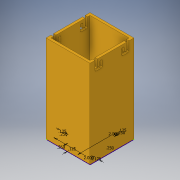
# Autodesk Inventor part: bateryHolder2.0
Saved by Autodesk Inventor 2017 (Build 210142000, 142)
## iProperties
Created: 2018-01-06
Part Number: bateryHolder2.0
Material: Generic
Document SubType Name: Modeling
Designer: User
Density: 1 g/cm^3
Appearance: Default(1)
Author: User
Autodesk Inventor part; units mm, degrees
ref_plane "YZ Plane" through (0, 0, 0) normal (1, 0, 0) x (0, 1, 0)
ref_plane "XZ Plane" through (0, 0, 0) normal (0, 1, 0) x (-1, 0, 0)
ref_plane "XY Plane" through (0, 0, 0) normal (0, 0, 1) x (1, 0, 0)
sketch "Sketch1" plane through (0, 0, 0) normal (0, 1, 0) x (-1, 0, 0)
  line L0 (0, 0) -> (50.8, 0)
  line L1 (50.8, 0) -> (50.8, -50.8)
  line L2 (50.8, -50.8) -> (0, -50.8)
  line L3 (0, -50.8) -> (0, 0)
  line L4 (53.975, 0) -> (53.975, 3.175)
  line L5 (53.975, 3.175) -> (50.8, 3.175)
  line L6 (-3.175, -50.8) -> (-3.175, -53.975)
  line L7 (-3.175, -53.975) -> (0, -53.975)
  line L8 (-3.175, -53.975) -> (53.975, -53.975)
  line L9 (53.975, -53.975) -> (53.975, 3.175)
  line L10 (53.975, 3.175) -> (-3.175, 3.175)
  line L11 (-3.175, 3.175) -> (-3.175, -53.975)
  line L12 (6.35, -6.35) -> (44.45, -6.35)
  line L13 (44.45, -6.35) -> (44.45, -44.45)
  line L14 (44.45, -44.45) -> (6.35, -44.45)
  line L15 (6.35, -44.45) -> (6.35, -6.35)
  dimension "d20" = 50.8
  dimension "d21" = 50.8
  dimension "d22" = 6.35
  dimension "d23" = 3.175
  dimension "d24" = 3.175
  dimension "d25" = 3.175
  dimension "d26" = 3.175
  dimension "d27" = 6.35
  dimension "d28" = 6.35
  dimension "d29" = 6.35
  constraints: 32 end point, 6 parallel, 3 horizontal, 3 perpendicular
  measures "d20" distance between parallel lines of L3 L1
  measures "d21" distance between parallel lines of L2 L0
  measures "d22" distance between parallel lines of L2 L14
  measures "d23" distance between parallel lines of L8 L2
  measures "d24" distance between parallel lines of L11 L3
  measures "d25" distance between parallel lines of L0 L10
  measures "d26" distance between parallel lines of L1 L9
  measures "d27" distance between parallel lines of L1 L13
  measures "d28" distance between parallel lines of L0 L12
  measures "d29" distance between parallel lines of L3 L15
extrude "Extrusion1" add sketch "Sketch1" along normal blind 114.3 contours L9 L8 L7 L6 L11 L10 L5 L4
sketch "Sketch2" plane through (3.175, 0, 3.175) normal (1, 0, 0) x (0, 0, -1)
  line L0 (3.175, 114.3) -> (53.975, 114.3) projected
  line L1 (50.8, 114.3) -> (47.625, 114.3)
  line L2 (47.625, 114.3) -> (47.625, 104.775)
  line L3 (49.0354, 101.6) -> (50.8, 101.6)
  line L4 (50.8, 101.6) -> (50.8, 114.3)
  line L5 (49.0354, 101.6) -> (41.275, 101.6)
  line L6 (41.275, 101.6) -> (41.275, 104.1556)
  line L7 (44.45, 104.775) -> (47.625, 104.775)
  line L8 (41.275, 101.6) -> (45.1552, 101.6)
  line L9 (44.45, 104.775) -> (44.45, 111.125)
  line L10 (44.45, 111.125) -> (41.275, 111.125)
  line L11 (41.275, 111.125) -> (41.275, 101.6)
  line L12 (57.15, 0) -> (57.15, 114.3) projected
  point P0 (3.175, 0)
  dimension "d10" = 3.175
  dimension "d11" = 6.35
  dimension "d12" = 9.525
  dimension "d13" = 3.175
  dimension "d14" = 3.175
  dimension "d15" = 3.175
  dimension "d16" = 12.7
  constraints: 22 end point, 5 parallel, 3 horizontal, 3 perpendicular, 1 point on line
  measures "d10" distance between parallel lines of L4 L2
  measures "d11" distance between parallel lines of L12 L4
  measures "d12" distance between parallel lines of L4 L11
  measures "d13" distance between parallel lines of L9 L11
  measures "d14" distance from line of L3.start L7
  measures "d15" distance between parallel lines of L0 L10
  measures "d16" distance between parallel lines of L0 L5
ref_plane "Work Plane1" through (-53.975, 0, -25.4) normal (0, 0, 1) x (1, 0, 0)
extrude "Extrusion3" cut sketch "Sketch2" against normal blind 3.175
ref_plane "Work Plane2" through (-25.4, 0, -53.975) normal (-1, 0, 0) x (0, 0, 1)
fillet "Fillet1" radius 1.5875 4 edges at (1.5875, 101.6, -38.1) (1.5875, 111.125, -38.1) (1.5875, 101.6, -47.625) (1.5875, 111.125, -41.275)
mirror "Mirror1" about plane through (-25.4, 0, -53.975) normal (-1, 0, 0) of "Extrusion3", "Fillet1"
mirror "Mirror2" about plane through (-53.975, 0, -25.4) normal (0, 0, 1) of "Extrusion3", "Fillet1", "Mirror1"
extrude "Extrusion4" cut sketch "Sketch1" along normal blind 3.175 contours L0 L1 L2 L3
extrude "Extrusion5" add sketch "Sketch1" against normal blind 3.175 contours L0 L1 L2 L3
ref_plane "Work Plane3" through (-53.975, 0, -25.4) normal (0, 0, 1) x (1, 0, 0)
body "Solid1"
